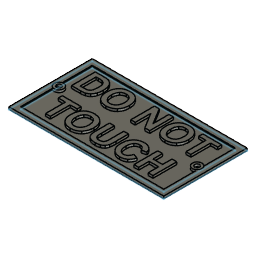
DoNotTouch (Autodesk Fusion 360 design; units mm, degrees)
Autodesk Fusion 360 part; units mm, degrees
note: some values were not read from the file. Set by a fixed rule: which face or edge a step refers to.
sketch "Sketch1" plane through (0, 0, 0) normal (0, 0, 1) x (1, 0, 0)
  line L0 (-5, 55) -> (115, 55)
  line L1 (115, 55) -> (115, -5)
  line L2 (115, -5) -> (-5, -5)
  line L3 (-5, -5) -> (-5, 55)
  line L4 (-10, 60) -> (120, 60)
  line L5 (120, 60) -> (120, -10)
  line L6 (120, -10) -> (-10, -10)
  line L7 (-10, -10) -> (-10, 60)
  constraint horizontal L0
  constraint vertical L1
  constraint horizontal L2
  constraint vertical L3
  constraint horizontal L4
  constraint vertical L5
  constraint horizontal L6
  constraint vertical L7
extrude "Extrude1" add sketch "Sketch1" along normal blind 1 contours L0 L1 L2 L3 makes body 1
extrude "Extrude2" add sketch "Sketch1" along normal blind 2 bodies 1
sketch "Sketch2" plane through (0, 0, 1) normal (0, 0, 1) x (-1, 0, 0)
  line L0 (5, 5) -> (-115, 5)
  line L1 (-115, 5) -> (-115, -55)
  line L2 (-115, -55) -> (5, -55)
  line L3 (5, -55) -> (5, 5)
  line L4 (5, 5) -> (-115, 5) construction
  line L5 (-115, 5) -> (-115, -55) construction
  line L6 (-115, -55) -> (5, -55) construction
  line L7 (5, -55) -> (5, 5) construction
  dimension "d7" = 20
  text T0 "DO NOT TOUCH" font "Arial" height 20 bold align centre middle in box 120 x 60 at (5, 5) x (-1, 0) y (0, -1) spacing 1 kerned
  constraint coincident L0.end
  constraint coincident L2.end
extrude "Extrude3" add sketch "Sketch2" along normal blind 3 text T0 bodies 1
sketch "Sketch3" plane through (0, 0, 1) normal (0, 0, 1) x (-1, 0, 0)
  spline S0 degree 3 poles (-22.6398, -9.2701) (-22.6648, -10.2165) (-22.7112, -11.9745) (-23.2877, -13.6337) (-23.5539, -14.3997) knots 0 0 0 0 0.281964 0.523808 0.523808 0.523808 0.523808
  spline S1 degree 3 poles (-23.5539, -14.3997) (-23.8026, -14.8966) (-24.3015, -15.8933) (-25.0438, -16.7248) (-25.4161, -17.1419) knots 0 0 0 0 0.165884 0.332772 0.332772 0.332772 0.332772
  spline S2 degree 3 poles (-25.4161, -17.1419) (-25.8121, -17.5176) (-26.583, -18.2491) (-27.5373, -18.7157) (-28.0014, -18.9427) knots 0 0 0 0 0.162679 0.316705 0.316705 0.316705 0.316705
  spline S3 degree 3 poles (-28.0014, -18.9427) (-28.6659, -19.1733) (-30.0614, -19.6576) (-31.5387, -19.7077) (-32.3124, -19.734) knots 0 0 0 0 0.209796 0.440523 0.440523 0.440523 0.440523
  spline S4 degree 3 poles (-32.3124, -19.734) (-33.692, -19.6399) (-36.3416, -19.4591) (-38.3997, -17.7912) (-39.3861, -16.9918) knots 0 0 0 0 0.403714 0.775328 0.775328 0.775328 0.775328
  spline S5 degree 3 poles (-39.3861, -16.9918) (-40.159, -15.9391) (-41.8187, -13.6787) (-41.9627, -10.8675) (-42.0396, -9.3656) knots 0 0 0 0 0.38345 0.823337 0.823337 0.823337 0.823337
  spline S6 degree 3 poles (-42.0396, -9.3656) (-41.9627, -7.8752) (-41.8188, -5.083) (-40.1736, -2.8352) (-39.4065, -1.7872) knots 0 0 0 0 0.436607 0.817949 0.817949 0.817949 0.817949
  spline S7 degree 3 poles (-39.4065, -1.7872) (-38.4264, -0.9898) (-36.3802, 0.675) (-33.7416, 0.8546) (-32.367, 0.9482) knots 0 0 0 0 0.369769 0.771942 0.771942 0.771942 0.771942
  spline S8 degree 3 poles (-32.367, 0.9482) (-30.9786, 0.8572) (-28.3244, 0.6833) (-26.2583, -0.9802) (-25.2728, -1.7735) knots 0 0 0 0 0.406149 0.776489 0.776489 0.776489 0.776489
  spline S9 degree 3 poles (-25.2728, -1.7735) (-24.5057, -2.812) (-22.8659, -5.0321) (-22.7183, -7.798) (-22.6398, -9.2701) knots 0 0 0 0 0.37901 0.810223 0.810223 0.810223 0.810223
  line L0 (-85.5593, 0.6071) -> (-85.5593, -19.3929)
  line L1 (-85.5593, -19.3929) -> (-89.5976, -19.3929)
  line L2 (-89.5976, -19.3929) -> (-89.5976, -11.5211)
  line L3 (-89.5976, -11.5211) -> (-97.5102, -11.5211)
  line L4 (-97.5102, -11.5211) -> (-97.5102, -19.3929)
  line L5 (-97.5102, -19.3929) -> (-101.5484, -19.3929)
  line L6 (-101.5484, -19.3929) -> (-101.5484, 0.6071)
  line L7 (-101.5484, 0.6071) -> (-97.5102, 0.6071)
  line L8 (-97.5102, 0.6071) -> (-97.5102, -8.1378)
  line L9 (-97.5102, -8.1378) -> (-89.5976, -8.1378)
  line L10 (-89.5976, -8.1378) -> (-89.5976, 0.6071)
  line L11 (-89.5976, 0.6071) -> (-85.5593, 0.6071)
  spline S10 degree 3 poles (-21.3438, -40.4843) (-21.3688, -41.4306) (-21.4151, -43.1887) (-21.9917, -44.8479) (-22.2578, -45.6139) knots 0 0 0 0 0.281964 0.523807 0.523807 0.523807 0.523807
  spline S11 degree 3 poles (-22.2578, -45.6139) (-22.5066, -46.1108) (-23.0055, -47.1075) (-23.7478, -47.939) (-24.1201, -48.3561) knots 0 0 0 0 0.165884 0.332772 0.332772 0.332772 0.332772
  spline S12 degree 3 poles (-24.1201, -48.3561) (-24.516, -48.7318) (-25.287, -49.4632) (-26.2412, -49.9299) (-26.7053, -50.1569) knots 0 0 0 0 0.162679 0.316705 0.316705 0.316705 0.316705
  spline S13 degree 3 poles (-26.7053, -50.1569) (-27.3699, -50.3875) (-28.7653, -50.8718) (-30.2426, -50.9219) (-31.0164, -50.9482) knots 0 0 0 0 0.209796 0.440523 0.440523 0.440523 0.440523
  spline S14 degree 3 poles (-31.0164, -50.9482) (-32.396, -50.854) (-35.0456, -50.6733) (-37.1036, -49.0054) (-38.09, -48.206) knots 0 0 0 0 0.403714 0.775328 0.775328 0.775328 0.775328
  spline S15 degree 3 poles (-38.09, -48.206) (-38.863, -47.1533) (-40.5227, -44.8929) (-40.6666, -42.0817) (-40.7435, -40.5798) knots 0 0 0 0 0.38345 0.823337 0.823337 0.823337 0.823337
  spline S16 degree 3 poles (-40.7435, -40.5798) (-40.6667, -39.0894) (-40.5227, -36.2972) (-38.8775, -34.0494) (-38.1105, -33.0014) knots 0 0 0 0 0.436607 0.817949 0.817949 0.817949 0.817949
  spline S17 degree 3 poles (-38.1105, -33.0014) (-37.1303, -32.2039) (-35.0841, -30.5392) (-32.4456, -30.3596) (-31.0709, -30.266) knots 0 0 0 0 0.369769 0.771942 0.771942 0.771942 0.771942
  spline S18 degree 3 poles (-31.0709, -30.266) (-29.6826, -30.357) (-27.0283, -30.5309) (-24.9622, -32.1944) (-23.9768, -32.9877) knots 0 0 0 0 0.406149 0.776489 0.776489 0.776489 0.776489
  spline S19 degree 3 poles (-23.9768, -32.9877) (-23.2097, -34.0262) (-21.5698, -36.2463) (-21.4223, -39.0122) (-21.3438, -40.4843) knots 0 0 0 0 0.37901 0.810223 0.810223 0.810223 0.810223
  line L12 (5, 5) -> (-115, 5)
  line L13 (-115, 5) -> (-115, -55)
  line L14 (-115, -55) -> (5, -55)
  line L15 (5, -55) -> (5, 5)
  spline S20 degree 3 poles (-71.0164, -40.4843) (-71.0413, -41.4306) (-71.0877, -43.1887) (-71.6642, -44.8479) (-71.9304, -45.6139) knots 0 0 0 0 0.281964 0.523808 0.523808 0.523808 0.523808
  spline S21 degree 3 poles (-71.9304, -45.6139) (-72.1791, -46.1108) (-72.6781, -47.1075) (-73.4204, -47.939) (-73.7926, -48.3561) knots 0 0 0 0 0.165884 0.332772 0.332772 0.332772 0.332772
  spline S22 degree 3 poles (-73.7926, -48.3561) (-74.1886, -48.7318) (-74.9595, -49.4632) (-75.9138, -49.9299) (-76.3779, -50.1569) knots 0 0 0 0 0.162679 0.316705 0.316705 0.316705 0.316705
  spline S23 degree 3 poles (-76.3779, -50.1569) (-77.0425, -50.3875) (-78.4379, -50.8718) (-79.9152, -50.9219) (-80.6889, -50.9482) knots 0 0 0 0 0.209797 0.440523 0.440523 0.440523 0.440523
  spline S24 degree 3 poles (-80.6889, -50.9482) (-82.0686, -50.854) (-84.7181, -50.6733) (-86.7762, -49.0054) (-87.7626, -48.206) knots 0 0 0 0 0.403715 0.775328 0.775328 0.775328 0.775328
  spline S25 degree 3 poles (-87.7626, -48.206) (-88.5356, -47.1533) (-90.1953, -44.8929) (-90.3392, -42.0817) (-90.4161, -40.5798) knots 0 0 0 0 0.38345 0.823337 0.823337 0.823337 0.823337
  spline S26 degree 3 poles (-90.4161, -40.5798) (-90.3393, -39.0894) (-90.1953, -36.2972) (-88.5501, -34.0494) (-87.7831, -33.0014) knots 0 0 0 0 0.436607 0.817949 0.817949 0.817949 0.817949
  spline S27 degree 3 poles (-87.7831, -33.0014) (-86.8029, -32.2039) (-84.7567, -30.5392) (-82.1182, -30.3596) (-80.7435, -30.266) knots 0 0 0 0 0.369769 0.771942 0.771942 0.771942 0.771942
  spline S28 degree 3 poles (-80.7435, -30.266) (-79.3552, -30.357) (-76.7009, -30.5309) (-74.6348, -32.1944) (-73.6494, -32.9877) knots 0 0 0 0 0.406149 0.776488 0.776488 0.776488 0.776488
  spline S29 degree 3 poles (-73.6494, -32.9877) (-72.8823, -34.0262) (-71.2424, -36.2463) (-71.0949, -39.0122) (-71.0164, -40.4843) knots 0 0 0 0 0.37901 0.810224 0.810224 0.810224 0.810224
  line L16 (-78.1651, -6.7462) -> (-82.0805, -5.5048)
  spline S30 degree 3 poles (-82.0805, -5.5048) (-81.7577, -4.5052) (-81.1538, -2.635) (-79.7428, -1.2746) (-79.0859, -0.6412) knots 0 0 0 0 0.309465 0.579038 0.579038 0.579038 0.579038
  spline S31 degree 3 poles (-79.0859, -0.6412) (-78.3145, -0.178) (-76.6823, 0.8019) (-74.7769, 0.8977) (-73.7722, 0.9482) knots 0 0 0 0 0.265781 0.562282 0.562282 0.562282 0.562282
  spline S32 degree 3 poles (-73.7722, 0.9482) (-72.5114, 0.8431) (-70.0341, 0.6367) (-68.1493, -0.9798) (-67.2237, -1.7735) knots 0 0 0 0 0.369216 0.72545 0.72545 0.72545 0.72545
  spline S33 degree 3 poles (-67.2237, -1.7735) (-66.4765, -2.8093) (-64.879, -5.0235) (-64.7354, -7.7594) (-64.6589, -9.2155) knots 0 0 0 0 0.375198 0.802107 0.802107 0.802107 0.802107
  spline S34 degree 3 poles (-64.6589, -9.2155) (-64.7292, -10.7445) (-64.8598, -13.5843) (-66.4865, -15.9017) (-67.2374, -16.9713) knots 0 0 0 0 0.448213 0.832451 0.832451 0.832451 0.832451
  spline S35 degree 3 poles (-67.2374, -16.9713) (-68.1845, -17.7769) (-70.1373, -19.438) (-72.6986, -19.6333) (-74.0177, -19.734) knots 0 0 0 0 0.363306 0.749143 0.749143 0.749143 0.749143
  spline S36 degree 3 poles (-74.0177, -19.734) (-75.166, -19.6597) (-77.37, -19.5173) (-79.1344, -18.1972) (-79.9795, -17.5648) knots 0 0 0 0 0.33693 0.646728 0.646728 0.646728 0.646728
  spline S37 degree 3 poles (-79.9795, -17.5648) (-80.4129, -17.0643) (-81.3503, -15.9817) (-81.7897, -14.6158) (-82.0259, -13.8813) knots 0 0 0 0 0.196597 0.425234 0.425234 0.425234 0.425234
  line L17 (-82.0259, -13.8813) -> (-78.0286, -12.9263)
  spline S38 degree 3 poles (-78.0286, -12.9263) (-77.8837, -13.413) (-77.6016, -14.3604) (-76.893, -15.0478) (-76.5484, -15.382) knots 0 0 0 0 0.149534 0.291043 0.291043 0.291043 0.291043
  spline S39 degree 3 poles (-76.5484, -15.382) (-76.1454, -15.6445) (-75.3145, -16.1859) (-74.3235, -16.2496) (-73.8131, -16.2824) knots 0 0 0 0 0.141775 0.292342 0.292342 0.292342 0.292342
  spline S40 degree 3 poles (-73.8131, -16.2824) (-73.1103, -16.2199) (-71.725, -16.0966) (-70.7065, -15.1517) (-70.2046, -14.6862) knots 0 0 0 0 0.205314 0.4047 0.4047 0.4047 0.4047
  spline S41 degree 3 poles (-70.2046, -14.6862) (-69.8028, -14.0057) (-68.8674, -12.4218) (-68.8372, -10.5712) (-68.8199, -9.5157) knots 0 0 0 0 0.233445 0.543365 0.543365 0.543365 0.543365
  spline S42 degree 3 poles (-68.8199, -9.5157) (-68.8316, -8.4047) (-68.8519, -6.4818) (-69.7886, -4.8164) (-70.1842, -4.1132) knots 0 0 0 0 0.32648 0.565084 0.565084 0.565084 0.565084
  spline S43 degree 3 poles (-70.1842, -4.1132) (-70.6765, -3.6437) (-71.6709, -2.6954) (-73.04, -2.5678) (-73.7312, -2.5034) knots 0 0 0 0 0.197969 0.399838 0.399838 0.399838 0.399838
  spline S44 degree 3 poles (-73.7312, -2.5034) (-74.2469, -2.5441) (-75.2669, -2.6247) (-76.0925, -3.2282) (-76.5007, -3.5266) knots 0 0 0 0 0.151897 0.300468 0.300468 0.300468 0.300468
  spline S45 degree 3 poles (-76.5007, -3.5266) (-76.8663, -3.9474) (-77.6787, -4.8823) (-77.9925, -6.0849) (-78.1651, -6.7462) knots 0 0 0 0 0.165076 0.366789 0.366789 0.366789 0.366789
  line L18 (-45.1637, -19.3929) -> (-49.2019, -19.3929)
  line L19 (-49.2019, -19.3929) -> (-49.2019, -8.5607)
  spline S46 degree 3 poles (-49.2019, -8.5607) (-49.1977, -7.8515) (-49.191, -6.7343) (-49.3089, -5.6238) (-49.352, -5.2183) knots 0 0 0 0 0.212516 0.334795 0.334795 0.334795 0.334795
  spline S47 degree 3 poles (-49.352, -5.2183) (-49.4672, -4.83) (-49.6962, -4.0582) (-50.2911, -3.5162) (-50.5866, -3.2469) knots 0 0 0 0 0.119037 0.236585 0.236585 0.236585 0.236585
  spline S48 degree 3 poles (-50.5866, -3.2469) (-50.9625, -3.0305) (-51.7851, -2.5568) (-52.7368, -2.5222) (-53.2538, -2.5034) knots 0 0 0 0 0.128212 0.280612 0.280612 0.280612 0.280612
  spline S49 degree 3 poles (-53.2538, -2.5034) (-53.7695, -2.5167) (-54.6949, -2.5405) (-55.4927, -3.0018) (-55.8458, -3.206) knots 0 0 0 0 0.15177 0.272352 0.272352 0.272352 0.272352
  spline S50 degree 3 poles (-55.8458, -3.206) (-56.1072, -3.4498) (-56.6192, -3.9275) (-56.8053, -4.6017) (-56.8963, -4.9318) knots 0 0 0 0 0.104955 0.205589 0.205589 0.205589 0.205589
  spline S51 degree 3 poles (-56.8963, -4.9318) (-56.9476, -5.385) (-57.0752, -6.5132) (-57.0742, -7.6492) (-57.0737, -8.3288) knots 0 0 0 0 0.136733 0.340397 0.340397 0.340397 0.340397
  line L20 (-57.0737, -8.3288) -> (-57.0737, -19.3929)
  line L21 (-57.0737, -19.3929) -> (-61.1119, -19.3929)
  line L22 (-61.1119, -19.3929) -> (-61.1119, -8.8881)
  spline S52 degree 3 poles (-61.1119, -8.8881) (-61.1137, -7.8616) (-61.1167, -6.1571) (-60.879, -4.4704) (-60.7844, -3.7995) knots 0 0 0 0 0.307408 0.510467 0.510467 0.510467 0.510467
  spline S53 degree 3 poles (-60.7844, -3.7995) (-60.6572, -3.3289) (-60.4104, -2.4165) (-59.8489, -1.657) (-59.5771, -1.2892) knots 0 0 0 0 0.144796 0.280736 0.280736 0.280736 0.280736
  spline S54 degree 3 poles (-59.5771, -1.2892) (-59.2492, -0.9615) (-58.5639, -0.2766) (-57.6831, 0.1293) (-57.2237, 0.3411) knots 0 0 0 0 0.137924 0.288303 0.288303 0.288303 0.288303
  spline S55 degree 3 poles (-57.2237, 0.3411) (-56.6617, 0.5177) (-55.4113, 0.9106) (-54.099, 0.9348) (-53.3765, 0.9482) knots 0 0 0 0 0.175847 0.391253 0.391253 0.391253 0.391253
  spline S56 degree 3 poles (-53.3765, 0.9482) (-52.5291, 0.9403) (-51.0461, 0.9266) (-49.6357, 0.4785) (-49.0314, 0.2865) knots 0 0 0 0 0.252418 0.44168 0.44168 0.44168 0.44168
  spline S57 degree 3 poles (-49.0314, 0.2865) (-48.571, 0.0581) (-47.6901, -0.3789) (-47.0143, -1.092) (-46.6917, -1.4325) knots 0 0 0 0 0.152781 0.292353 0.292353 0.292353 0.292353
  spline S58 degree 3 poles (-46.6917, -1.4325) (-46.4314, -1.782) (-45.9283, -2.4574) (-45.6794, -3.2614) (-45.5593, -3.6494) knots 0 0 0 0 0.129644 0.250558 0.250558 0.250558 0.250558
  spline S59 degree 3 poles (-45.5593, -3.6494) (-45.4447, -4.3574) (-45.1726, -6.037) (-45.167, -7.7396) (-45.1637, -8.7244) knots 0 0 0 0 0.214882 0.509728 0.509728 0.509728 0.509728
  line L23 (-45.1637, -8.7244) -> (-45.1637, -19.3929)
  line L24 (-11.3984, 0.6071) -> (-11.3984, -16.0095)
  line L25 (-11.3984, -16.0095) -> (-5.4638, -16.0095)
  line L26 (-5.4638, -16.0095) -> (-5.4638, -19.3929)
  line L27 (-5.4638, -19.3929) -> (-21.3574, -19.3929)
  line L28 (-21.3574, -19.3929) -> (-21.3574, -16.0095)
  line L29 (-21.3574, -16.0095) -> (-15.4366, -16.0095)
  line L30 (-15.4366, -16.0095) -> (-15.4366, 0.6071)
  line L31 (-15.4366, 0.6071) -> (-11.3984, 0.6071)
  line L32 (-98.0696, -30.6071) -> (-98.0696, -47.2237)
  line L33 (-98.0696, -47.2237) -> (-92.1351, -47.2237)
  line L34 (-92.1351, -47.2237) -> (-92.1351, -50.6071)
  line L35 (-92.1351, -50.6071) -> (-108.0287, -50.6071)
  line L36 (-108.0287, -50.6071) -> (-108.0287, -47.2237)
  line L37 (-108.0287, -47.2237) -> (-102.1078, -47.2237)
  line L38 (-102.1078, -47.2237) -> (-102.1078, -30.6071)
  line L39 (-102.1078, -30.6071) -> (-98.0696, -30.6071)
  line L40 (-51.6985, -30.6071) -> (-51.6985, -50.6071)
  line L41 (-51.6985, -50.6071) -> (-55.6276, -50.6071)
  line L42 (-55.6276, -50.6071) -> (-63.8131, -37.251)
  line L43 (-63.8131, -37.251) -> (-63.8131, -50.6071)
  line L44 (-63.8131, -50.6071) -> (-67.5648, -50.6071)
  line L45 (-67.5648, -50.6071) -> (-67.5648, -30.6071)
  line L46 (-67.5648, -30.6071) -> (-63.513, -30.6071)
  line L47 (-63.513, -30.6071) -> (-55.4502, -43.6494)
  line L48 (-55.4502, -43.6494) -> (-55.4502, -30.6071)
  line L49 (-55.4502, -30.6071) -> (-51.6985, -30.6071)
  line L50 (-1.9713, -50.6071) -> (-9.352, -50.6071)
  spline S60 degree 3 poles (-9.352, -50.6071) (-10.0883, -50.6031) (-11.3704, -50.5962) (-12.6245, -50.3359) (-13.1583, -50.2251) knots 0 0 0 0 0.220194 0.38337 0.38337 0.38337 0.38337
  spline S61 degree 3 poles (-13.1583, -50.2251) (-13.7235, -50.0191) (-14.8523, -49.6077) (-15.7334, -48.7911) (-16.1733, -48.3834) knots 0 0 0 0 0.178518 0.356482 0.356482 0.356482 0.356482
  spline S62 degree 3 poles (-16.1733, -48.3834) (-16.5694, -47.9093) (-17.3837, -46.9347) (-17.8459, -45.7511) (-18.0832, -45.1432) knots 0 0 0 0 0.184038 0.378336 0.378336 0.378336 0.378336
  spline S63 degree 3 poles (-18.0832, -45.1432) (-18.2739, -44.4338) (-18.6896, -42.8868) (-18.721, -41.2839) (-18.7381, -40.4161) knots 0 0 0 0 0.219581 0.478795 0.478795 0.478795 0.478795
  spline S64 degree 3 poles (-18.7381, -40.4161) (-18.7202, -39.6448) (-18.6867, -38.2004) (-18.303, -36.8084) (-18.1241, -36.1596) knots 0 0 0 0 0.230389 0.431502 0.431502 0.431502 0.431502
  spline S65 degree 3 poles (-18.1241, -36.1596) (-17.8587, -35.478) (-17.3508, -34.1738) (-16.4245, -33.1262) (-15.9823, -32.6262) knots 0 0 0 0 0.217462 0.416091 0.416091 0.416091 0.416091
  spline S66 degree 3 poles (-15.9823, -32.6262) (-15.5844, -32.2987) (-14.7345, -31.5989) (-13.6967, -31.2276) (-13.1446, -31.03) knots 0 0 0 0 0.153416 0.327759 0.327759 0.327759 0.327759
  spline S67 degree 3 poles (-13.1446, -31.03) (-12.6261, -30.9071) (-11.4521, -30.6288) (-10.2445, -30.6149) (-9.5703, -30.6071) knots 0 0 0 0 0.159395 0.360901 0.360901 0.360901 0.360901
  line L51 (-9.5703, -30.6071) -> (-1.9713, -30.6071)
  line L52 (-1.9713, -30.6071) -> (-1.9713, -50.6071)
  circle A0 centre (3, -25) radius 2
  circle A1 centre (3, -25) radius 4
  circle A2 centre (-113, -25) radius 2
  circle A3 centre (-113, -25) radius 4
  constraint concentric A0 A1
  constraint concentric A2 A3
extrude "Extrude4" add sketch "Sketch3" along normal blind 4 separate body contours L15 A1 | L15 A1 | L13 A3 | L13 A3 makes body 2 at (111.7261, 21.2083, 2.3333) makes body 3 at (-6.9801, 24.6017, 3.6667)
extrude "Extrude5" cut 10 faces at (3.3174, 42.8126, 4) (39.2561, 39.3606, 4) (52.9491, 41.6212, 4) (88.9287, 39.3606, 4) (100.7617, 36.146, 4) (100.2024, 8.9745, 4) (66.1315, 10.5651, 4) (58.4197, 12.2033, 4) (40.5522, 8.1464, 4) (14.0905, 10.4707, 4) along direction (0, 0, -1) blind 1 on bodies 1 bodies 1
extrude "Extrude6" cut 2 faces at (111.9726, 28.1617, 5) (-6.3184, 24.8013, 5) along direction (0, 0, -1) blind 2 on bodies 2 3 bodies 2 3
equation "d8 = 'DO NOT TOUCH'"
